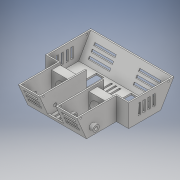
# Autodesk Inventor part: Main_Chassi_2
Saved by Autodesk Inventor 2018.2 (Build 222227000, 227)
## iProperties
Created: 2018-08-11
Part Number: Main_Chassi_2
Material: Generic
Document SubType Name: Modeling
Designer: mateu
Density: 1 g/cm^3
Appearance: Default
Author: mateu
Autodesk Inventor part; units mm, degrees
ref_plane "YZ Plane" through (0, 0, 0) normal (1, 0, 0) x (0, 1, 0)
sketch "Sketch1" plane through (0, 0, 0) normal (0, 0, 1) x (1, 0, 0)
  line L0 (0, 0) -> (110, 0)
  line L1 (110, 0) -> (110, 56)
  line L2 (0, 56) -> (0, 0)
  line L3 (110, 56) -> (133, 56)
  line L4 (0, 56) -> (-23, 56)
  line L5 (55, 116) -> (25, 116)
  line L6 (25, 116) -> (55, 116)
  line L7 (55, 116) -> (85, 116)
  line L8 (133, 56) -> (133, 116)
  line L9 (133, 116) -> (85, 116)
  line L10 (-23, 56) -> (-23, 116)
  line L11 (-23, 116) -> (25, 116)
  dimension "d0" = 110
  dimension "d1" = 56
  dimension "d2" = 23
  dimension "d3" = 23
  dimension "d7" = 30
  dimension "d8" = 30
  dimension "d17" = 60
  constraints: 24 end point, 4 horizontal, 2 collinear, 2 perpendicular, 2 vertical, 1 parallel, 1 point on line
  measures "d0" distance of L2.start L1.end
  measures "d1" distance of L1.end L0.end
  measures "d2" distance of L1.end L3.end
  measures "d3" distance of L2.start L4.end
  measures "d7" distance of L5.start L5.end
  measures "d8" distance of L5.start L7.end
  measures "d17" distance of L4.end L10.end
extrude "Extrusion1" add sketch "Sketch1" along normal blind 3
sketch "Sketch3" plane through (0, 0, 3) normal (0, 0, 1) x (1, 0, 0)
  line L0 (110, 56) -> (133, 56) projected
  line L1 (110, 0) -> (110, 56)
  line L2 (110, 56) -> (133, 56)
  line L3 (133, 56) -> (133, 116) projected
  line L4 (133, 56) -> (133, 116)
  line L5 (-23, 116) -> (-23, 56) projected
  line L6 (-23, 116) -> (-23, 56)
  line L7 (-23, 56) -> (0, 56)
  line L8 (0, 56) -> (0, 0) projected
  line L9 (0, 56) -> (0, 0)
  line L10 (2.4, 58.4) -> (-20.6, 58.4)
  line L11 (130.6, 58.4) -> (107.6, 58.4)
  line L12 (107.6, 58.4) -> (107.6, 2.4)
  line L13 (2.4, 2.4) -> (2.4, 58.4)
  line L14 (2.4, 2.4) -> (2.4, 0)
  line L15 (107.6, 2.4) -> (107.6, 0)
  line L16 (2.4, 0) -> (0, 0)
  line L17 (107.6, 0) -> (110, 0)
  line L18 (-23, 116) -> (-20.6, 116)
  line L19 (-23, 116) -> (-23, 56) projected
  line L20 (133, 56) -> (133, 116) projected
  line L21 (130.6, 116) -> (133, 116)
  line L22 (-20.6, 58.4) -> (-20.6, 116)
  line L23 (133, 116) -> (-23, 116) projected
  line L24 (130.6, 58.4) -> (130.6, 116)
  dimension "d18" = 2.4
  constraints: 36 end point, 5 equal length, 4 perpendicular, 1 point on line, 1 other
  measures "d18" distance between parallel lines of L7 L10
extrude "Extrusion3" add sketch "Sketch3" along normal blind 39
sketch "Sketch4" plane through (133, 56, 0) normal (1, 0, 0) x (0, 0, -1)
  line L0 (0, 60) -> (-42, 60) projected
  line L1 (0, 60) -> (-42, 60)
  line L2 (-42, 60) -> (-42, 85)
  line L3 (-42, 85) -> (0, 60)
  point P0 (0, -56)
  dimension "d21" = 25
  constraints: 6 end point, 1 collinear, 1 perpendicular
  measures "d21" distance of L0.end L2.end
extrude "Extrusion4" add sketch "Sketch4" against normal blind 2.4
sketch "Sketch5" plane through (-23, 56, 0) normal (-1, 0, 0) x (0, 0, 1)
  line L0 (0, 60) -> (42, 60) projected
  line L1 (42, 0) -> (42, 85) projected
  line L2 (42, 60) -> (42, 85)
  line L3 (3, 60) -> (0, 60) projected
  line L4 (42, 85) -> (0, 60)
  line L5 (0, 60) -> (42, 60)
  point P0 (0, -56)
  constraints: 6 end point, 2 collinear
extrude "Extrusion5" add sketch "Sketch5" against normal blind 2.4
sketch "Sketch6" plane through (130.6, 58.4, 3) normal (-1, 0, 0) x (0, 0, 1)
  line L0 (0, 57.6) -> (-3, 57.6) projected
  line L1 (-3, 57.6) -> (0, 57.6)
  line L2 (39, 82.6) -> (-3, 57.6) projected
  line L3 (39, 82.6) -> (39, 80.2)
  line L4 (39, 0) -> (39, 82.6) projected
  line L5 (39, 80.2) -> (0, 57.6)
  line L6 (-3, 57.6) -> (39, 82.6) projected
  line L7 (39, 82.6) -> (-3, 57.6)
  point P0 (-3, -58.4)
  dimension "d26" = 2.4
  constraints: 8 end point, 2 collinear, 1 point on line
  measures "d26" distance of L2.start L3.end
extrude "Extrusion6" add sketch "Sketch6" along normal blind 153.6
sketch "Sketch7" plane through (0, 0, 0) normal (-1, 0, 0) x (0, 0, 1)
  line L0 (0, 0) -> (0, 56) projected
  line L1 (0, 0) -> (42, -17.8979)
  line L2 (42, 0) -> (42, 58.4) projected
  line L3 (42, -17.8979) -> (42, 0)
  line L4 (42, 0) -> (42, 56) projected
  line L5 (0, 0) -> (42, 0)
  constraints: 6 end point, 1 collinear, 1 horizontal
extrude "Extrusion7" add sketch "Sketch7" against normal blind 2.4
sketch "Sketch8" plane through (110, 0, 0) normal (1, 0, 0) x (0, 0, -1)
  line L0 (-42, 58.4) -> (-42, 0) projected
  line L1 (-42, 0) -> (0, 0)
  line L2 (-3, 0) -> (-42, 0) projected
  line L3 (-42, -17.8979) -> (0, 0) projected
  line L4 (0, 0) -> (-42, -17.8979)
  line L5 (-42, -17.8979) -> (-42, 0)
  line L6 (-42, 58.4) -> (-42, 0) projected
  constraints: 6 end point, 3 collinear
extrude "Extrusion8" add sketch "Sketch8" against normal blind 2.4
sketch "Sketch10" plane through (0, 0, 3) normal (0, 0, 1) x (1, 0, 0)
  line L0 (40, 0) -> (40, 70)
  line L1 (133, 116) -> (-23, 116) projected
  line L2 (40, 70) -> (37.6, 70)
  line L3 (37.6, 70) -> (37.6, 0)
  line L4 (37.6, 0) -> (40, 0)
  line L5 (2.4, 0) -> (107.6, 0) projected
  line L6 (70, 0) -> (72.4, 0)
  line L7 (72.4, 0) -> (72.4, 70)
  line L8 (72.4, 70) -> (70, 70)
  line L9 (70, 70) -> (70, 0)
  point P0 (0, 0)
  dimension "d37" = 70
  dimension "d38" = 2.4
  dimension "d39" = 2.4
  constraints: 16 end point, 3 perpendicular, 2 parallel, 1 collinear, 1 horizontal
  measures "d37" distance of L0.start L0.end
  measures "d38" distance of L0.end L2.end
  measures "d39" distance of L8.end L7.end
extrude "Extrusion9" add sketch "Sketch10" along normal blind 39
sketch "Sketch11" plane through (37.6, 0, 3) normal (-1, 0, 0) x (0, 0, 1)
  line L0 (0, 0) -> (39, 0) projected
  line L1 (-3, 0) -> (39, 0)
  line L2 (39, 58.4) -> (39, -17.8979) projected
  line L3 (39, 0) -> (39, -17.8979)
  line L4 (39, -17.8979) -> (-3, 0)
  constraints: 6 end point, 1 horizontal, 1 perpendicular
extrude "Extrusion10" add sketch "Sketch11" against normal blind 2.4
sketch "Sketch12" plane through (70, 0, 3) normal (-1, 0, 0) x (0, 0, 1)
  line L0 (0, 0) -> (39, 0) projected
  line L1 (-3, 0) -> (39, 0)
  line L2 (39, 70) -> (39, -17.8979) projected
  line L3 (39, 0) -> (39, -17.8979)
  line L4 (39, -17.8979) -> (-3, 0)
  constraints: 6 end point, 1 collinear, 1 perpendicular
extrude "Extrusion11" add sketch "Sketch12" against normal blind 2.4
sketch "Sketch13" plane through (72.4, 0, 3) normal (1, 0, 0) x (0, 0, -1)
  line L0 (-39, 70) -> (-39, -17.8979) projected
  line L1 (-39, -17.8979) -> (-39, -15.4979)
  line L2 (0, 70) -> (0, 0) projected
  line L3 (-39, -15.4979) -> (0, 0)
  line L4 (0, 0) -> (3, 0)
  line L5 (-39, -17.8979) -> (3, 0) projected
  line L6 (3, 0) -> (-39, -17.8979)
  dimension "d46" = 2.4
  constraints: 8 end point, 1 collinear, 1 perpendicular, 1 point on line
  measures "d46" distance of L0.end L1.end
extrude "Extrusion12" add sketch "Sketch13" along normal blind 36
sketch "Sketch14" plane through (2.4, 0, 3) normal (1, 0, 0) x (0, 0, -1)
  line L0 (-39, 58.4) -> (-39, -17.8979) projected
  line L1 (-39, -17.8979) -> (-39, -15.4979)
  line L2 (-39, -15.4979) -> (0, 0)
  line L3 (0, 0) -> (3, 0) projected
  line L4 (0, 0) -> (3, 0)
  line L5 (-39, -17.8979) -> (3, 0) projected
  line L6 (3, 0) -> (-39, -17.8979)
  dimension "d49" = 2.4
  constraints: 8 end point, 2 collinear, 1 point on line
  measures "d49" distance of L0.end L1.end
extrude "Extrusion13" add sketch "Sketch14" along normal blind 36
sketch "Sketch15" plane through (70, 0, 3) normal (-1, 0, 0) x (0, 0, 1)
  line L0 (-3, 0) -> (3.5492, 0)
  line L1 (3.5492, 0) -> (3.5492, -2.7909)
  line L2 (-3, 0) -> (39, -17.8979) projected
  line L3 (3.5492, -2.7909) -> (-3, 0)
  constraints: 6 end point, 1 collinear, 1 horizontal, 1 perpendicular
extrude "Extrusion14" add sketch "Sketch15" along normal blind 30
sketch "Sketch17" plane through (110, 56, 42) normal (1, 0, 0) x (0, 0, -1)
  circle A0 centre (27, -45) radius 21.5
  line L0 (42, -56) -> (42, 0) projected
  line L1 (42, 0) -> (0, 0) projected
  circle A1 centre (27, -45) radius 6
  dimension "d61" = 43
  dimension "d62" = 15
  dimension "d63" = 45
  dimension "d64" = 12
  constraints: 2 centre point, 1 coincident
  measures "d61" diameter of A0
  measures "d62" distance from line of L0 A0.centre
  measures "d63" distance from line of L1 A0.centre
  measures "d64" diameter of A1
extrude "Extrusion16" add sketch "Sketch17" along normal blind 7 contours A1
sketch "Sketch18" plane through (117, 11, 15) normal (1, 0, 0) x (0, 0, -1)
  circle A0 centre (0, 0) radius 2.85
  point P0 (15, -11)
  dimension "d67" = 5.7
  constraints: 1 centre point
  measures "d67" diameter of A0
extrude "Extrusion17" cut sketch "Sketch18" against normal blind 650
sketch "Sketch19" plane through (0, 56, 0) normal (-1, 0, 0) x (0, 0, 1)
  circle A0 centre (15, -45) radius 21.5
  line L0 (0, 0) -> (42, 0) projected
  line L1 (0, 0) -> (0, -56) projected
  circle A1 centre (15, -45) radius 2.85 projected
  circle A2 centre (15, -45) radius 6
  circle A3 centre (15, -45) radius 2.625
  dimension "d70" = 43
  dimension "d71" = 45
  dimension "d72" = 15
  dimension "d73" = 12
  dimension "d74" = 5.25
  constraints: 3 centre point, 2 coincident
  measures "d70" diameter of A0
  measures "d71" distance from line of L0 A0.centre
  measures "d72" distance from line of L1 A0.centre
  measures "d73" diameter of A2
  measures "d74" diameter of A3
extrude "Extrusion18" add sketch "Sketch19" along normal blind 7 contours A2
sketch "Sketch27" plane through (0, 0, 3) normal (0, 0, 1) x (1, 0, 0)
  line L0 (70, 0) -> (40, 0) projected
  line L1 (60, 115) -> (50, 115) projected
  line L2 (53.5, 0.7671) -> (56.5, 0.7671)
  line L3 (56.5, 0.7671) -> (56.5, 110.7671)
  line L4 (56.5, 110.7671) -> (53.5, 110.7671)
  line L5 (53.5, 110.7671) -> (53.5, 0.7671)
  line L6 (61.5, 0.7671) -> (64.5, 0.7671)
  line L7 (64.5, 0.7671) -> (64.5, 110.7671)
  line L8 (64.5, 110.7671) -> (61.5, 110.7671)
  line L9 (61.5, 110.7671) -> (61.5, 0.7671)
  line L10 (48.5, 0.7671) -> (45.5, 0.7671)
  line L11 (45.5, 0.7671) -> (45.5, 110.7671)
  line L12 (45.5, 110.7671) -> (48.5, 110.7671)
  line L13 (48.5, 110.7671) -> (48.5, 0.7671)
  line L14 (70, 70) -> (70, -17.8979) projected
  point P0 (0, 0)
  dimension "d170" = 3
  dimension "d171" = 110
  dimension "d172" = 3
  dimension "d173" = 3
  dimension "d174" = 110
  dimension "d175" = 13.5
  dimension "d176" = 5
  dimension "d177" = 5
  constraints: 24 end point, 6 parallel, 3 horizontal, 3 perpendicular, 3 point on line
  measures "d170" distance of L4.end L3.end
  measures "d171" distance of L3.end L2.end
  measures "d172" distance of L8.end L7.end
  measures "d173" distance of L11.end L12.end
  measures "d174" distance of L10.end L11.end
  measures "d175" distance between parallel lines of L3 L14
  measures "d176" distance between parallel lines of L3 L9
  measures "d177" distance between parallel lines of L5 L13
extrude "Extrusion26" cut sketch "Sketch27" against normal blind 4
sketch "Sketch31" plane through (0, 0, 3) normal (0, 0, 1) x (1, 0, 0)
  line L0 (2.4, 58.4) -> (2.4, 0) projected
  line L1 (37.6, 0) -> (37.6, 70) projected
  line L2 (2.4, 47) -> (37.6, 47)
  line L3 (37.6, 47) -> (37.6, 42)
  line L4 (37.6, 42) -> (2.4, 42)
  line L5 (2.4, 42) -> (2.4, 47)
  line L6 (107.6, 58.4) -> (107.6, -15.4979) projected
  line L7 (72.4812, 47) -> (107.6, 47)
  line L8 (107.6, 47) -> (107.6, 42)
  line L9 (107.6, 42) -> (72.4812, 42)
  line L10 (72.4812, 42) -> (72.4812, 47)
  line L11 (2.4, 0) -> (37.6, 0) projected
  point P0 (0, 0)
  dimension "d206" = 5
  dimension "d209" = 42
  constraints: 16 end point, 5 point on line, 4 parallel, 2 horizontal, 2 perpendicular
  measures "d206" distance of L2.end L3.end
  measures "d209" distance between parallel lines of L11 L4
extrude "Extrusion30" add sketch "Sketch31" along normal blind 34 contours L2 L1 L4 L0 | L6 L9 L10 L7
sketch "Sketch33" plane through (72.4812, 47, 3) normal (0, 1, 0) x (1, 0, 0)
  line L0 (35.1188, -34) -> (0, -34) projected
  line L1 (35.1188, -34) -> (-0.0812, -34)
  line L2 (-0.0812, -34) -> (-0.0812, 0)
  line L3 (-0.0812, 0) -> (35.1188, 0)
  line L4 (35.1188, 0) -> (35.1188, -34)
  line L5 (-34.8812, -34) -> (-70.0812, -34) projected
  line L6 (-70.0812, 0) -> (-34.8812, 0) projected
  line L7 (-70.0812, -34) -> (-34.8812, -34)
  line L8 (-34.8812, -34) -> (-34.8812, 0)
  line L9 (-34.8812, 0) -> (-70.0812, 0)
  line L10 (-70.0812, 0) -> (-70.0812, -34)
  point P0 (-72.4812, 3)
  constraints: 16 end point, 4 parallel, 2 horizontal, 2 perpendicular
extrude "Extrusion33" add sketch "Sketch33" along normal blind 11
sketch "Sketch32" plane through (2.4, 42, 3) normal (0, -1, 0) x (1, 0, 0)
  line L0 (35.2, 0) -> (0, 0) projected
  line L1 (35.2, 34) -> (35.2, 0) projected
  line L2 (70.0812, 0) -> (70.0812, 34) projected
  line L3 (105.2, 0) -> (70.0812, 0) projected
  circle A0 centre (20.2, 12) radius 13.125
  circle A1 centre (85.0812, 12) radius 13.125
  point P0 (-2.4, -3)
  dimension "d228" = 26.25
  dimension "d229" = 26.25
  constraints: 2 centre point
  measures "d228" diameter of A0
  measures "d229" diameter of A1
extrude "Extrusion34" cut sketch "Sketch32" along normal blind 5 and the other way blind 20
sketch "Sketch34" plane through (0, 0, 3) normal (0, 0, 1) x (1, 0, 0)
  line L0 (27.9165, 37) -> (17.2835, 37) projected
  line L1 (10, 106) -> (100, 106) projected
  line L2 (2.4, 58) -> (37.6, 58) projected
  line L3 (22.6, 58) -> (15.6, 58)
  line L4 (15.6, 58) -> (15.6, 113)
  line L5 (15.6, 113) -> (22.6, 113)
  line L6 (22.6, 113) -> (29.6, 113)
  line L7 (29.6, 113) -> (29.6, 58)
  line L8 (29.6, 58) -> (22.6, 58)
  line L9 (82.1647, 37) -> (92.7978, 37) projected
  line L10 (87.4812, 58) -> (80.4812, 58)
  line L11 (72.4, 58) -> (107.6, 58) projected
  line L12 (80.4812, 58) -> (80.4812, 113)
  line L13 (80.4812, 113) -> (94.4812, 113)
  line L14 (94.4812, 113) -> (94.4812, 58)
  point P0 (0, 0)
  dimension "d236" = 7
  dimension "d237" = 55
  dimension "d238" = 7
  dimension "d239" = 7
  dimension "d240" = 55
  dimension "d241" = 14
  constraints: 20 end point, 5 perpendicular, 4 point on line, 2 horizontal, 2 parallel
  measures "d236" distance of L4.end L5.end
  measures "d237" distance of L3.end L4.end
  measures "d238" distance of L7.end L8.end
  measures "d239" distance of L10.start L10.end
  measures "d240" distance of L10.end L12.end
  measures "d241" distance of L12.end L13.end
extrude "Extrusion35" cut sketch "Sketch34" against normal blind 23
sketch "Sketch35" plane through (-23, 56, 0) normal (-1, 0, 0) x (0, 0, 1)
  line L0 (32.4094, 49.5058) -> (12.4094, 49.5058)
  line L1 (12.4094, 49.5058) -> (12.4094, 45.5058)
  line L2 (12.4094, 45.5058) -> (32.4094, 45.5058)
  line L3 (32.4094, 45.5058) -> (32.4094, 49.5058)
  line L4 (32.4094, 40.246) -> (12.4094, 40.246)
  line L5 (12.4094, 40.246) -> (12.4094, 36.246)
  line L6 (12.4094, 36.246) -> (32.4094, 36.246)
  line L7 (32.4094, 36.246) -> (32.4094, 40.246)
  line L8 (32.4094, 30.8459) -> (12.4094, 30.8459)
  line L9 (12.4094, 30.8459) -> (12.4094, 26.8459)
  line L10 (12.4094, 26.8459) -> (32.4094, 26.8459)
  line L11 (32.4094, 26.8459) -> (32.4094, 30.8459)
  line L12 (32.4094, 22.0069) -> (12.4094, 22.0069)
  line L13 (12.4094, 22.0069) -> (12.4094, 18.0069)
  line L14 (12.4094, 18.0069) -> (32.4094, 18.0069)
  line L15 (32.4094, 18.0069) -> (32.4094, 22.0069)
  point P0 (0, -56)
  dimension "d244" = 20
  dimension "d245" = 4
  dimension "d246" = 4
  dimension "d247" = 4
  dimension "d248" = 4
  constraints: 32 end point, 8 parallel, 4 horizontal, 4 perpendicular, 4 point on line
  measures "d244" distance of L0.start L0.end
  measures "d245" distance of L2.end L0.start
  measures "d246" distance of L5.end L4.end
  measures "d247" distance of L9.end L8.end
  measures "d248" distance of L13.end L12.end
extrude "Extrusion36" cut sketch "Sketch35" against normal blind 156
sketch "Sketch36" plane through (37.6, 70, 3) normal (-1, 0, 0) x (0, 0, 1)
  circle A0 centre (36, -80.8979) radius 1.5
  line L0 (39, 0) -> (39, -85.4979) projected
  point P0 (-3, -70)
  point P1 (39, -87.8979)
  dimension "d251" = 3
  dimension "d252" = 3
  dimension "d253" = 7
  constraints: 1 centre point
  measures "d251" diameter of A0
  measures "d252" distance from line of L0 A0.centre
  measures "d253" vertical distance of point (39, -87.898) A0.centre
extrude "Extrusion37" cut sketch "Sketch36" along normal blind 50 and the other way blind 100
ref_plane "Work Plane1" through (0, -25, 0) normal (0, 1, 0) x (-1, 0, 0)
sketch "Sketch37" plane through (0, -25, 0) normal (0, 1, 0) x (-1, 0, 0)
  line L0 (-7, 34.7873) -> (-32, 34.7873)
  line L1 (-32, 34.7873) -> (-32, 30.7873)
  line L2 (-32, 30.7873) -> (-7, 30.7873)
  line L3 (-7, 30.7873) -> (-7, 34.7873)
  line L4 (-7, 25.4142) -> (-32, 25.4142)
  line L5 (-32, 25.4142) -> (-32, 21.4142)
  line L6 (-32, 21.4142) -> (-7, 21.4142)
  line L7 (-7, 21.4142) -> (-7, 25.4142)
  line L8 (-7, 17.312) -> (-32, 17.312)
  line L9 (-32, 17.312) -> (-32, 13.312)
  line L10 (-32, 13.312) -> (-7, 13.312)
  line L11 (-7, 13.312) -> (-7, 17.312)
  line L12 (-40, 42) -> (-40, 6.5492) projected
  line L13 (-78, 34.7873) -> (-103, 34.7873)
  line L14 (-103, 34.7873) -> (-103, 30.7873)
  line L15 (-103, 30.7873) -> (-78, 30.7873)
  line L16 (-78, 30.7873) -> (-78, 34.7873)
  line L17 (-78, 25.4142) -> (-103, 25.4142)
  line L18 (-103, 25.4142) -> (-103, 21.4142)
  line L19 (-103, 21.4142) -> (-78, 21.4142)
  line L20 (-78, 21.4142) -> (-78, 25.4142)
  line L21 (-78, 17.312) -> (-103, 17.312)
  line L22 (-103, 17.312) -> (-103, 13.312)
  line L23 (-103, 13.312) -> (-78, 13.312)
  line L24 (-78, 13.312) -> (-78, 17.312)
  line L25 (-70, 6.5492) -> (-70, 42) projected
  point P0 (0, 0)
  dimension "d257" = 25
  dimension "d258" = 4
  dimension "d259" = 4
  dimension "d260" = 4
  dimension "d261" = 8
  dimension "d262" = 25
  dimension "d263" = 4
  dimension "d264" = 4
  dimension "d265" = 8
  dimension "d268" = 25
  constraints: 48 end point, 12 parallel, 7 point on line, 6 horizontal, 6 perpendicular
  measures "d257" distance of L2.end L1.end
  measures "d258" distance of L1.end L0.end
  measures "d259" distance of L5.end L4.end
  measures "d260" distance of L9.end L8.end
  measures "d261" distance between parallel lines of L12 L1
  measures "d262" distance of L15.end L14.end
  measures "d263" distance of L14.end L13.end
  measures "d264" distance of L22.end L21.end
  measures "d265" distance between parallel lines of L25 L16
  measures "d268" distance of L22.end L23.end
extrude "Extrusion38" cut sketch "Sketch37" along normal blind 40
ref_plane "Work Plane2" through (0, 150, 0) normal (0, 1, 0) x (-1, 0, 0)
sketch "Sketch38" plane through (0, 150, 0) normal (0, 1, 0) x (-1, 0, 0)
  line L0 (-133, 0) -> (-133, 42) projected
  line L1 (23, 0) -> (23, 42) projected
  line L2 (-133, 42) -> (23, 42)
  line L3 (23, 42) -> (23, 0)
  line L4 (23, 0) -> (-133, 0)
  line L5 (-133, 0) -> (-133, 42)
  line L6 (-130.6, 42) -> (20.6, 42) projected
  line L7 (-55, 42) -> (-55, 0)
  line L8 (-117, 31.8563) -> (-77, 31.8563)
  line L9 (-77, 31.8563) -> (-77, 27.8563)
  line L10 (-77, 27.8563) -> (-117, 27.8563)
  line L11 (-117, 27.8563) -> (-117, 31.8563)
  line L12 (-117, 23.4331) -> (-77, 23.4331)
  line L13 (-77, 23.4331) -> (-77, 19.4331)
  line L14 (-77, 19.4331) -> (-117, 19.4331)
  line L15 (-117, 19.4331) -> (-117, 23.4331)
  line L16 (-117, 14.542) -> (-77, 14.542)
  line L17 (-77, 14.542) -> (-77, 10.542)
  line L18 (-77, 10.542) -> (-117, 10.542)
  line L19 (-117, 10.542) -> (-117, 14.542)
  line L20 (-33, 31.8563) -> (7, 31.8563)
  line L21 (7, 31.8563) -> (7, 27.8563)
  line L22 (7, 27.8563) -> (-33, 27.8563)
  line L23 (-33, 27.8563) -> (-33, 31.8563)
  line L24 (-33, 23.4331) -> (7, 23.4331)
  line L25 (7, 23.4331) -> (7, 19.4331)
  line L26 (7, 19.4331) -> (-33, 19.4331)
  line L27 (-33, 19.4331) -> (-33, 23.4331)
  line L28 (-33, 14.542) -> (7, 14.542)
  line L29 (7, 14.542) -> (7, 10.542)
  line L30 (7, 10.542) -> (-33, 10.542)
  line L31 (-33, 10.542) -> (-33, 14.542)
  point P0 (0, 0)
  dimension "d270" = 40
  dimension "d271" = 4
  dimension "d272" = 4
  dimension "d273" = 4
  dimension "d274" = 40
  dimension "d275" = 4
  dimension "d276" = 22
  dimension "d277" = 22
  dimension "d293" = 40
  constraints: 58 end point, 14 parallel, 12 point on line, 7 horizontal, 7 perpendicular, 2 midpoint
  measures "d270" distance of L9.end L10.end
  measures "d271" distance of L8.end L9.end
  measures "d272" distance of L12.end L13.end
  measures "d273" distance of L16.end L17.end
  measures "d274" distance of L21.end L22.end
  measures "d275" distance of L28.end L29.end
  measures "d276" distance between parallel lines of L7 L9
  measures "d277" distance between parallel lines of L7 L23
  measures "d293" distance of L29.end L30.end
extrude "Extrusion39" cut sketch "Sketch38" against normal blind 40 contours L8 L9 L10 L11 | L12 L13 L14 L15 | L16 L17 L18 L19 | L20 L21 L22 L23 | L24 L25 L26 L27 | L28 L29 L30 L31
sketch "Sketch39" plane through (72.4, 70, 42) normal (1, 0, 0) x (0, 0, -1)
  circle A0 centre (27, -59) radius 2.85 projected
  circle A1 centre (27, -59) radius 5
  point P0 (42, -70)
  dimension "d280" = 10
  constraints: 1 centre point, 1 coincident
  measures "d280" diameter of A1
extrude "Extrusion40" add sketch "Sketch39" along normal blind 5
sketch "Sketch40" plane through (37.6, 70, 3) normal (-1, 0, 0) x (0, 0, 1)
  circle A0 centre (12, -59) radius 2.85 projected
  circle A1 centre (12, -59) radius 5
  point P0 (-3, -70)
  dimension "d283" = 10
  constraints: 1 centre point, 1 coincident
  measures "d283" diameter of A1
extrude "Extrusion41" add sketch "Sketch40" along normal blind 5
sketch "Sketch41" plane through (0, 0, 3) normal (0, 0, 1) x (1, 0, 0)
  line L0 (7.6, 33.6721) -> (30.6, 33.6721)
  line L1 (30.6, 33.6721) -> (30.6, 3.6721)
  line L2 (30.6, 3.6721) -> (7.6, 3.6721)
  line L3 (7.6, 3.6721) -> (7.6, 33.6721)
  line L4 (79.4, 33.6721) -> (102.4, 33.6721)
  line L5 (102.4, 33.6721) -> (102.4, 3.6721)
  line L6 (102.4, 3.6721) -> (79.4, 3.6721)
  line L7 (79.4, 3.6721) -> (79.4, 33.6721)
  line L8 (72.4, 70) -> (72.4, -15.4979) projected
  line L9 (37.6, 70) -> (37.6, -15.4979) projected
  point P0 (0, 0)
  dimension "d286" = 23
  dimension "d287" = 30
  dimension "d288" = 23
  dimension "d289" = 7
  dimension "d290" = 7
  constraints: 16 end point, 4 parallel, 2 horizontal, 2 perpendicular, 2 point on line
  measures "d286" distance of L1.end L2.end
  measures "d287" distance of L0.end L1.end
  measures "d288" distance of L5.end L6.end
  measures "d289" distance between parallel lines of L8 L7
  measures "d290" distance between parallel lines of L1 L9
extrude "Extrusion42" cut sketch "Sketch41" against normal blind 5
sketch "Sketch42" plane through (133, 56, 42) normal (1, 0, 0) x (0, 0, -1)
  circle A0 centre (3, 75.0681) radius 1.5
  line L0 (0, 0) -> (0, 85) projected
  line L1 (42, 60) -> (0, 85) projected
  point P0 (42, -56)
  dimension "d294" = 3
  dimension "d295" = 3
  dimension "d296" = 7
  constraints: 1 centre point
  measures "d294" diameter of A0
  measures "d295" distance from line of L0 A0.centre
  measures "d296" distance from line of L1 A0.centre
extrude "Extrusion43" cut sketch "Sketch42" against normal blind 156
body "Solid1"
